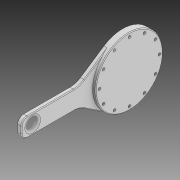
# Autodesk Inventor part: testweight_arm
Saved by Autodesk Inventor 2020 (Build 240168000, 168)
## iProperties
Created: 2021-03-20
Part Number: testweight_arm
Material: Generic
Document SubType Name: Modeling
Designer: DDeGo
Density: 1 g/cm^3
Appearance: Default
Author: DDeGo
Autodesk Inventor part; units mm, degrees
ref_plane "YZ Plane" through (0, 0, 0) normal (1, 0, 0) x (0, 1, 0)
ref_plane "XZ Plane" through (0, 0, 0) normal (0, 1, 0) x (-1, 0, 0)
ref_plane "XY Plane" through (0, 0, 0) normal (0, 0, 1) x (1, 0, 0)
sketch "Sketch1" plane through (0, 0, 0) normal (1, 0, 0) x (0, 1, 0)
  line L0 (0, 0) -> (0, 125) construction
  arc A0 (-37.480621, 24.903876) -> (37.480621, 24.903876) centre (0, 0) ccw
  circle A1 centre (0, 0) radius 40 construction
  circle A2 centre (0, 40) radius 1.75
  circle A3 centre (-20, 34.641016) radius 1.75
  circle A4 centre (-34.641016, 20) radius 1.75
  circle A5 centre (-40, 0) radius 1.75
  circle A6 centre (-34.641016, -20) radius 1.75
  circle A7 centre (-20, -34.641016) radius 1.75
  circle A8 centre (0, -40) radius 1.75
  circle A9 centre (20, -34.641016) radius 1.75
  circle A10 centre (34.641016, -20) radius 1.75
  circle A11 centre (40, 0) radius 1.75
  circle A12 centre (34.641016, 20) radius 1.75
  circle A13 centre (20, 34.641016) radius 1.75
  line L1 (-37.480621, 24.903876) -> (-12.5, 62.5)
  line L2 (-12.5, 62.5) -> (12.5, 62.5) construction
  line L3 (12.5, 62.5) -> (37.480621, 24.903876)
  line L4 (12.5, 62.5) -> (12.5, 132)
  line L5 (4.5, 140) -> (-4.5, 140)
  line L6 (-12.5, 132) -> (-12.5, 62.5)
  line L7 (0, 140) -> (0, 125) construction
  circle A14 centre (0, 125) radius 7.5
  arc A15 (12.5, 132) -> (4.5, 140) centre (4.5, 132) ccw
  arc A16 (-4.5, 140) -> (-12.5, 132) centre (-4.5, 132) ccw
  line L8 (0, 0) -> (0, -45) construction
  point P0 (0, 62.5)
  point P1 (12.5, 140)
  point P2 (-12.5, 140)
  dimension "d3" = 80
  dimension "d0" = 45
  dimension "d1" = 125
  dimension "d2" = 3.5
  dimension "d6" = 360
  dimension "d8" = 25
  dimension "d9" = 15
  dimension "d10" = 15
  dimension "d11" = 8
  dimension "d16" = 185
  constraints: 20 end point, 16 centre point, 7 point on circle, 6 tangent, 5 point on line, 4 vertical, 3 midpoint, 2 coincident, 2 perpendicular, 1 equal radius, 1 horizontal, 1 vertical alignment, 27 other
  measures "d0" radius of A0
  measures "d1" distance of L0.start L0.end
  measures "d2" diameter of A2
  measures "d8" distance of point (12.5, 140) point (-12.5, 140)
  measures "d9" diameter of A14
  measures "d10" distance from line of A14.centre L5
  measures "d11" radius of A15
  measures "d16" distance of L7.start L8.end
extrude "Extrusion1" add sketch "Sketch1" along normal blind 10
sketch "Sketch2" plane through (10, 0, 0) normal (1, 0, 0) x (0, 0, -1)
  arc A0 (-24.903876, -37.480621) -> (-24.903876, 37.480621) centre (0, 0) ccw
  circle A1 centre (0, 0) radius 45
  circle A2 centre (0, 0) radius 183.297075
  point P0 (-24.903876, -37.480621)
  constraints: 2 coincident, 1 centre point, 3 other
extrude "Extrusion2" cut sketch "Sketch2" against normal blind 4
fillet "Fillet1" radius 25 2 edges at (3, 12.5, 62.5) (3, -12.5, 62.5)
fillet "Fillet2" radius 3 2 edges at (0, -7.5, 125) (6, -7.5, 125)
chamfer "Chamfer1" distance 1 angle 45 20 edges at (0, 27.079, 40.5584) (0, 13.5671, 62.8222) (0, 12.5, 101.0242) (0, 10.1569, 137.6569) (0, 0, 140) (0, -10.1569, 137.6569) (0, -12.5, 101.0242) (0, -13.5671, 62.8222) (0, -27.079, 40.5584) (0, 0, -45) (6, 13.5671, 62.8222) (6, 27.079, 40.5584) (6, 12.5, 101.0242) (6, 10.1569, 137.6569) (6, 0, 140) (6, -10.1569, 137.6569) (6, -12.5, 101.0242) (6, -13.5671, 62.8222) (6, -27.079, 40.5584) (10, 37.4806, -24.9039)
body "Solid1"
